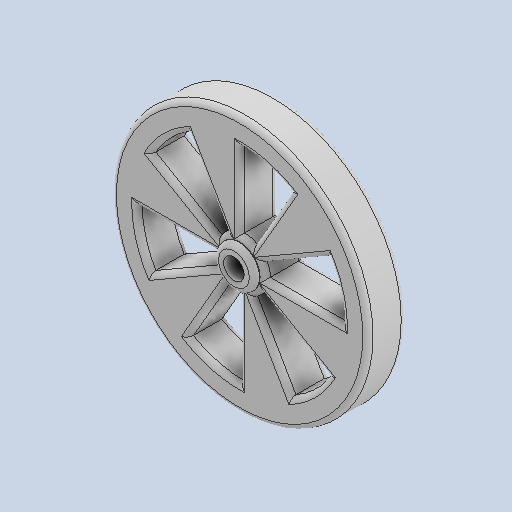
# Autodesk Inventor part: wheel final
Saved by Autodesk Inventor 2022 (Build 260153000, 153)
## iProperties
Created: 2021-07-02
Part Number: wheel final
Material: Generic
Document SubType Name: Modeling
Designer: HP
Density: 1 g/cm^3
Appearance: Default
Author: HP
Autodesk Inventor part; units mm, degrees
ref_plane "YZ Plane" through (0, 0, 0) normal (1, 0, 0) x (0, 1, 0)
ref_plane "XZ Plane" through (0, 0, 0) normal (0, 1, 0) x (-1, 0, 0)
ref_plane "XY Plane" through (0, 0, 0) normal (0, 0, 1) x (1, 0, 0)
sketch "Sketch1" plane through (0, 0, 0) normal (0, 0, 1) x (1, 0, 0)
  circle A0 centre (0, 0) radius 50
  dimension "d0" = 100
  constraints: 1 centre point, 1 coincident
  measures "d0" diameter of A0
extrude "Extrusion1" add sketch "Sketch1" along normal blind 15
sketch "Sketch2" plane through (0, 0, 15) normal (0, 0, 1) x (1, 0, 0)
  circle A0 centre (0, 0) radius 40
  arc A1 (10, 0) -> (8.6603, 5) centre (0, 0) ccw
  line L0 (10, 0) -> (40, 0)
  line L1 (8.6603, 5) -> (34.641, 20)
  line L2 (0, 0) -> (40, 0) construction
  point P0 (34.641, 20)
  dimension "d3" = 80
  dimension "d4" = 20
  dimension "d5" = 40
  dimension "d6" = 30
  constraints: 6 end point, 2 coincident, 2 horizontal, 2 point on circle, 1 centre point, 1 point on line, 3 other
  measures "d4" diameter of A1
  measures "d5" distance of L2.start L1.end
  measures "d6" angle of L2 L1
extrude "Extrusion2" cut sketch "Sketch2" against normal blind 15 contours L0 A1 L1 A0 picked at (29.7974, 2.3153)
pattern_circular "Circular Pattern1" count 6 over 360 about axis through (0, 0, 0) along (0, 0, 1) of "Extrusion2"
fillet "Fillet1" radius 2 50 edges at (-50, 0, 15) (-21.6506, 12.5, 15) (-28.2843, 28.2843, 15) (-12.5, 21.6506, 15) (0, 25, 15) (-7.0711, 7.0711, 15) (-9.6593, -2.5882, 15) (-21.6506, -12.5, 15) (-12.5, -21.6506, 15) (-2.5882, -9.6593, 15) (0, -25, 15) (12.5, -21.6506, 15) (7.0711, -7.0711, 15) (21.6506, -12.5, 15) (25, 0, 15) (9.6593, 2.5882, 15) (21.6506, 12.5, 15) (-25, 0, 15) (12.5, 21.6506, 15) (2.5882, 9.6593, 15) (10.3528, 38.637, 15) (38.637, 10.3528, 15) (28.2843, -28.2843, 15) (-10.3528, -38.637, 15) (-38.637, -10.3528, 15) (21.6506, -12.5, 0) (7.0711, -7.0711, 0) (12.5, -21.6506, 0) (28.2843, -28.2843, 0) (25, 0, 0) (38.637, 10.3528, 0) (21.6506, 12.5, 0) (9.6593, 2.5882, 0) (2.5882, 9.6593, 0) (0, 25, 0) (12.5, 21.6506, 0) (10.3528, 38.637, 0) (-50, 0, 0) (-28.2843, 28.2843, 0) (-12.5, 21.6506, 0) (-21.6506, 12.5, 0) (-7.0711, 7.0711, 0) (-9.6593, -2.5882, 0) (-21.6506, -12.5, 0) (-25, 0, 0) (-38.637, -10.3528, 0) (-10.3528, -38.637, 0) (-12.5, -21.6506, 0) (0, -25, 0) (-2.5882, -9.6593, 0)
sketch "Sketch3" plane through (0, 0, 15) normal (0, 0, 1) x (1, 0, 0)
  arc A0 (2.1409, -7.7082) -> (7.7082, -2.1409) centre (0, 0) ccw projected
  circle A1 centre (0, 0) radius 8
  point P0 (2.1409, -7.7082)
  constraints: 1 coincident, 3 other
extrude "Extrusion3" add sketch "Sketch3" along normal blind 2.2
fillet "Fillet2" radius 2 1 edges at (-2.1409, 7.7082, 17.2)
sketch "Sketch4" plane through (0, 0, 17.2) normal (0, 0, 1) x (1, 0, 0)
  circle A0 centre (0, 0) radius 4
  dimension "d16" = 8
  constraints: 1 centre point, 1 coincident
  measures "d16" diameter of A0
extrude "Extrusion4" cut sketch "Sketch4" against normal through all
body "Solid1"
